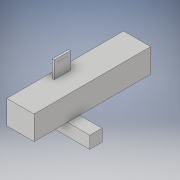
# Autodesk Inventor part: CLB_056_4StagePlaceholder
Saved by Autodesk Inventor 2018.3 (Build 223284000, 284)
## iProperties
Created: 2020-02-16
Part Number: CLB_056_4StagePlaceholder
Material: Generic
Document SubType Name: Modeling
Designer: 21vogecale
Density: 1 g/cm^3
Appearance: Default
Author: 21vogecale
Autodesk Inventor part; units mm, degrees
ref_plane "YZ Plane" through (0, 0, 0) normal (1, 0, 0) x (0, 1, 0)
ref_plane "XZ Plane" through (0, 0, 0) normal (0, 1, 0) x (-1, 0, 0)
ref_plane "XY Plane" through (0, 0, 0) normal (0, 0, 1) x (1, 0, 0)
sketch "Sketch1" plane through (0, 0, 0) normal (0, 1, 0) x (-1, 0, 0)
  line L0 (-53.3048, 57.4444) -> (73.6952, 57.4444)
  line L1 (73.6952, 57.4444) -> (73.6952, -488.6556)
  line L2 (73.6952, -488.6556) -> (-53.3048, -488.6556)
  line L3 (-53.3048, -488.6556) -> (-53.3048, 57.4444)
  point P0 (0, 0)
  dimension "d0" = 127
  dimension "d1" = 546.1
  constraints: 8 end point, 2 parallel, 1 horizontal, 1 perpendicular
  measures "d0" distance of L0.start L0.end
  measures "d1" distance of L0.end L1.end
extrude "Extrusion1" add sketch "Sketch1" along normal blind 111.76
sketch "Sketch2" plane through (0, 111.76, 0) normal (0, 1, 0) x (1, 0, 0)
  line L0 (-38.6432, 129.0678) -> (-48.2952, 129.0678)
  line L1 (-48.2952, 129.0678) -> (-48.2952, 206.0298)
  line L2 (-48.2952, 206.0298) -> (-38.6432, 206.0298)
  line L3 (-38.6432, 206.0298) -> (-38.6432, 129.0678)
  line L4 (53.3048, -57.4444) -> (53.3048, 488.6556) projected
  line L5 (-73.6952, 488.6556) -> (-73.6952, -57.4444) projected
  line L6 (-73.6952, -57.4444) -> (53.3048, -57.4444) projected
  point P0 (0, 0)
  dimension "d4" = 9.652
  dimension "d5" = 76.962
  dimension "d8" = 25.4
  dimension "d9" = 186.5122
  constraints: 8 end point, 2 parallel, 1 horizontal, 1 perpendicular
  measures "d4" distance of L1.end L2.end
  measures "d5" distance between parallel lines of L2 L0
  measures "d8" distance between parallel lines of L5 L1
  measures "d9" distance between parallel lines of L6 L0
extrude "Extrusion2" add sketch "Sketch2" along normal blind 79.375
sketch "Sketch3" plane through (-38.6432, 111.76, -129.0678) normal (1, 0, 0) x (0, 0, -1)
  line L0 (16.1079, 65.0185) -> (71.5479, 65.0185) construction
  line L1 (71.5479, 65.0185) -> (71.5479, 29.0665) construction
  line L2 (71.5479, 29.0665) -> (16.1079, 29.0665) construction
  line L3 (16.1079, 29.0665) -> (16.1079, 65.0185) construction
  point P0 (-129.0678, -111.76)
  constraints: 2 other
sketch "Sketch4" plane through (0, 0, 0) normal (0, -1, 0) x (1, 0, 0)
  line L0 (-19.5932, -155.9156) -> (158.2068, -155.9156)
  line L1 (158.2068, -155.9156) -> (158.2068, -98.7656)
  line L2 (158.2068, -98.7656) -> (-19.5932, -98.7656)
  line L3 (-19.5932, -98.7656) -> (-19.5932, -155.9156)
  line L4 (-73.6952, -488.6556) -> (53.3048, -488.6556) projected
  line L5 (-73.6952, 57.4444) -> (-73.6952, -488.6556) projected
  point P0 (0, 0)
  dimension "d13" = 332.74
  dimension "d14" = 57.15
  dimension "d15" = 54.102
  dimension "d16" = 177.8
  constraints: 8 end point, 2 parallel, 1 horizontal, 1 perpendicular
  measures "d13" distance between parallel lines of L4 L0
  measures "d14" distance of L2.end L0.start
  measures "d15" distance between parallel lines of L5 L3
  measures "d16" distance of L0.start L0.end
extrude "Extrusion3" add sketch "Sketch4" along normal blind 57.15
sketch "Sketch5" plane through (158.2068, 0, -155.9156) normal (0, 0, -1) x (-1, 0, 0)
  line L0 (25.6026, -7.1293) -> (89.7659, -7.1293) construction
  line L1 (89.7659, -7.1293) -> (89.7659, -41.3497) construction
  line L2 (89.7659, -41.3497) -> (25.6026, -41.3497) construction
  line L3 (25.6026, -41.3497) -> (25.6026, -7.1293) construction
  point P0 (158.2068, 0)
  constraints: 2 other
body "Solid1"
